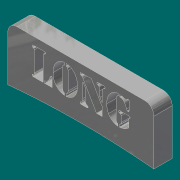
# Autodesk Inventor part: A1-19010-100-04 Tab - LONG
Saved by Autodesk Inventor 2017 SP1 (Build 210196100, 196)
## iProperties
Created: 2014-10-23
Part Number: A1-19010-100-04 Tab - LONG
Material: Steel, Mild
Description: 4" x 1 1/2" x 1/2" PLATE, A516 Gr.70
Document SubType Name: Modeling
Designer: Graeme_Van_Dongen
Density: 7.86 g/cm^3
Appearance: Steel
Mass: 297.606 g
Surface Area: 145.562 cm^2
Volume: 37.8634 cm^3
Author: Graeme_Van_Dongen
Autodesk Inventor part; units mm, degrees
ref_plane "YZ Plane" through (0, 0, 0) normal (1, 0, 0) x (0, 1, 0)
ref_plane "XZ Plane" through (0, 0, 0) normal (0, 1, 0) x (-1, 0, 0)
ref_plane "XY Plane" through (0, 0, 0) normal (0, 0, 1) x (1, 0, 0)
sketch "Sketch1" plane through (0, 0, 0) normal (0, 0, 1) x (1, 0, 0)
  arc A0 (50.8, 543.7321) -> (-50.8, 543.7321) centre (0, 0) ccw
  line L0 (50.8, 543.7321) -> (50.8, 581.8321)
  line L1 (50.8, 581.8321) -> (-50.8, 581.8321)
  line L2 (-50.8, 581.8321) -> (-50.8, 543.7321)
  point P0 (0, 581.8321)
  dimension "d0" = 101.6
  dimension "d1" = 38.1
  dimension "d2" = 546.1
  constraints: 6 end point, 2 parallel, 2 point on circle, 1 centre point, 1 coincident, 1 midpoint, 1 perpendicular, 1 vertical, 1 vertical alignment
  measures "d0" distance of L0.end L1.end
  measures "d1" distance of L0.start L0.end
  measures "d2" radius of A0
extrude "Extrusion1" add sketch "Sketch1" along normal mid plane 12.7
sketch "Sketch2" plane through (0, 0, 6.35) normal (0, 0, 1) x (1, 0, 0)
  line L0 (-46.29, 576.8125) -> (46.3638, 576.8125) construction
  line L1 (46.3638, 576.8125) -> (46.3638, 557.0018) construction
  line L2 (46.3638, 557.0018) -> (-46.29, 557.0018) construction
  line L3 (-46.29, 557.0018) -> (-46.29, 576.8125) construction
  line L4 (-26.3305, 557.3821) -> (-32.5482, 557.3821)
  line L5 (-32.5482, 557.3821) -> (-32.912, 557.3821)
  spline S0 degree 2 poles (-32.912, 557.3821) (-33.4081, 557.3821) (-33.9538, 557.7625) (-33.9538, 558.1097) knots 0 0 0 1 2 2 2
  spline S1 degree 2 poles (-33.9538, 558.1097) (-33.9538, 558.672) (-33.3915, 558.8539) knots 0 0 0 1 1 1
  spline S2 degree 2 poles (-33.3915, 558.8539) (-32.9285, 559.0192) (-32.7797, 559.0854) (-32.697, 559.2177) knots 0 0 0 1 2 2 2
  spline S3 degree 2 poles (-32.697, 559.2177) (-32.5316, 559.4326) (-32.5316, 559.9287) knots 0 0 0 1 1 1
  line L6 (-32.5316, 559.9287) -> (-32.5316, 573.8855)
  spline S4 degree 2 poles (-32.5316, 573.8855) (-32.5316, 574.3816) (-32.697, 574.5966) knots 0 0 0 1 1 1
  spline S5 degree 2 poles (-32.697, 574.5966) (-32.7797, 574.7289) (-32.9285, 574.795) (-33.3915, 574.9438) knots 0 0 0 1 2 2 2
  spline S6 degree 2 poles (-33.3915, 574.9438) (-33.9538, 575.1257) (-33.9538, 575.7045) knots 0 0 0 1 1 1
  spline S7 degree 2 poles (-33.9538, 575.7045) (-33.9538, 576.0518) (-33.4081, 576.4321) (-32.912, 576.4321) knots 0 0 0 1 2 2 2
  line L7 (-32.912, 576.4321) -> (-32.5482, 576.4321)
  line L8 (-32.5482, 576.4321) -> (-26.3139, 576.4321)
  line L9 (-26.3139, 576.4321) -> (-25.8344, 576.4321)
  spline S8 degree 2 poles (-25.8344, 576.4321) (-25.2225, 576.4321) (-24.9579, 576.2667) knots 0 0 0 1 1 1
  spline S9 degree 2 poles (-24.9579, 576.2667) (-24.5941, 576.0352) (-24.5941, 575.6714) knots 0 0 0 1 1 1
  spline S10 degree 2 poles (-24.5941, 575.6714) (-24.5941, 575.0596) (-25.2721, 574.9108) knots 0 0 0 1 1 1
  spline S11 degree 2 poles (-25.2721, 574.9108) (-25.8178, 574.7785) (-26.0163, 574.6958) (-26.1155, 574.58) knots 0 0 0 1 2 2 2
  spline S12 degree 2 poles (-26.1155, 574.58) (-26.3305, 574.3154) (-26.3305, 573.7863) knots 0 0 0 1 1 1
  line L10 (-26.3305, 573.7863) -> (-26.3305, 557.3821)
  line L11 (-25.1895, 557.3821) -> (-25.1895, 558.9531)
  spline S13 degree 2 poles (-25.1895, 558.9531) (-24.5115, 559.0688) (-23.7177, 559.383) (-23.3539, 559.6641) knots 0 0 0 1 2 2 2
  spline S14 degree 2 poles (-23.3539, 559.6641) (-22.7586, 560.1272) (-21.7829, 561.7477) (-21.4853, 562.7399) knots 0 0 0 1 2 2 2
  spline S15 degree 2 poles (-21.4853, 562.7399) (-21.2538, 563.5006) (-20.89, 563.9967) (-20.5262, 563.9967) knots 0 0 0 1 2 2 2
  spline S16 degree 2 poles (-20.5262, 563.9967) (-20.1293, 563.9967) (-19.9474, 563.6825) knots 0 0 0 1 1 1
  spline S17 degree 2 poles (-19.9474, 563.6825) (-19.8647, 563.5171) (-19.8647, 563.0541) knots 0 0 0 1 1 1
  line L12 (-19.8647, 563.0541) -> (-19.8647, 557.3821)
  line L13 (-19.8647, 557.3821) -> (-25.1895, 557.3821)
  line L14 (-10.2405, 575.3076) -> (-10.2405, 576.8125)
  spline S18 degree 2 poles (-10.2405, 576.8125) (-8.7357, 576.7463) (-6.2387, 575.6549) (-5.1638, 574.5966) knots 0 0 0 1 2 2 2
  spline S19 degree 2 poles (-5.1638, 574.5966) (-2.3195, 571.8184) (-2.3195, 566.8906) knots 0 0 0 1 1 1
  spline S20 degree 2 poles (-2.3195, 566.8906) (-2.3195, 562.0454) (-5.0315, 559.3334) knots 0 0 0 1 1 1
  spline S21 degree 2 poles (-5.0315, 559.3334) (-7.1316, 557.2498) (-10.2405, 557.0018) knots 0 0 0 1 1 1
  line L15 (-10.2405, 557.0018) -> (-10.2405, 558.5397)
  spline S22 degree 2 poles (-10.2405, 558.5397) (-9.8767, 558.6223) (-9.4798, 558.8869) (-9.3145, 559.135) knots 0 0 0 1 2 2 2
  spline S23 degree 2 poles (-9.3145, 559.135) (-8.9341, 559.7138) (-8.9341, 560.8713) knots 0 0 0 1 1 1
  line L16 (-8.9341, 560.8713) -> (-8.9341, 573.3398)
  spline S24 degree 2 poles (-8.9341, 573.3398) (-8.9341, 574.0839) (-9.1822, 574.5139) knots 0 0 0 1 1 1
  spline S25 degree 2 poles (-9.1822, 574.5139) (-9.3475, 574.8115) (-9.8105, 575.1423) (-10.2405, 575.3076) knots 0 0 0 1 2 2 2
  spline S26 degree 2 poles (-11.3815, 575.3076) (-12.0926, 575.0431) (-12.6714, 574.1832) (-12.6714, 573.3398) knots 0 0 0 1 2 2 2
  line L17 (-12.6714, 573.3398) -> (-12.6714, 560.8713)
  spline S27 degree 2 poles (-12.6714, 560.8713) (-12.6714, 559.6476) (-12.3406, 559.135) knots 0 0 0 1 1 1
  spline S28 degree 2 poles (-12.3406, 559.135) (-12.076, 558.7216) (-11.3815, 558.5397) knots 0 0 0 1 1 1
  line L18 (-11.3815, 558.5397) -> (-11.3815, 557.0018)
  spline S29 degree 2 poles (-11.3815, 557.0018) (-14.4738, 557.2498) (-16.574, 559.3334) knots 0 0 0 1 1 1
  spline S30 degree 2 poles (-16.574, 559.3334) (-19.2859, 562.0454) (-19.2859, 566.8906) knots 0 0 0 1 1 1
  spline S31 degree 2 poles (-19.2859, 566.8906) (-19.2859, 569.3214) (-17.8473, 573.2406) (-16.4417, 574.5966) knots 0 0 0 1 2 2 2
  spline S32 degree 2 poles (-16.4417, 574.5966) (-15.3668, 575.6549) (-12.8863, 576.7463) (-11.3815, 576.8125) knots 0 0 0 1 2 2 2
  line L19 (-11.3815, 576.8125) -> (-11.3815, 575.3076)
  line L20 (7.3047, 576.4321) -> (14.7296, 563.5337)
  line L21 (14.7296, 563.5337) -> (14.7296, 557.3821)
  line L22 (14.7296, 557.3821) -> (10.9262, 557.3821)
  line L23 (10.9262, 557.3821) -> (1.4508, 573.7036)
  spline S33 degree 2 poles (1.4508, 573.7036) (1.1366, 574.2493) (0.7397, 574.6627) (0.4421, 574.7619) knots 0 0 0 1 2 2 2
  line L24 (0.4421, 574.7619) -> (-0.0871, 574.9604)
  spline S34 degree 2 poles (-0.0871, 574.9604) (-0.3021, 575.0265) (-0.5501, 575.3903) (-0.5501, 575.6053) knots 0 0 0 1 2 2 2
  spline S35 degree 2 poles (-0.5501, 575.6053) (-0.5501, 575.8533) (-0.3021, 576.2502) (-0.0871, 576.3329) knots 0 0 0 1 2 2 2
  spline S36 degree 2 poles (-0.0871, 576.3329) (0.1444, 576.4321) (1.2027, 576.4321) knots 0 0 0 1 1 1
  line L25 (1.2027, 576.4321) -> (7.3047, 576.4321)
  line L26 (1.4508, 571.5208) -> (2.9225, 569.0734)
  line L27 (2.9225, 569.0734) -> (2.9225, 561.5989)
  spline S37 degree 2 poles (2.9225, 561.5989) (2.9225, 560.6233) (3.584, 559.3665) (4.295, 558.9531) knots 0 0 0 1 2 2 2
  line L28 (4.295, 558.9531) -> (4.7085, 558.7216)
  spline S38 degree 2 poles (4.7085, 558.7216) (5.0723, 558.5066) (5.0723, 558.0932) knots 0 0 0 1 1 1
  spline S39 degree 2 poles (5.0723, 558.0932) (5.0723, 557.779) (4.8077, 557.564) knots 0 0 0 1 1 1
  spline S40 degree 2 poles (4.8077, 557.564) (4.5762, 557.3821) (3.8816, 557.3821) knots 0 0 0 1 1 1
  line L29 (3.8816, 557.3821) -> (0.6736, 557.3821)
  spline S41 degree 2 poles (0.6736, 557.3821) (-0.5997, 557.3821) (-0.5997, 558.1097) knots 0 0 0 1 1 1
  spline S42 degree 2 poles (-0.5997, 558.1097) (-0.5997, 558.3578) (-0.3352, 558.6554) (0.1113, 558.9035) knots 0 0 0 1 2 2 2
  spline S43 degree 2 poles (0.1113, 558.9035) (1.4508, 559.6476) (1.4508, 561.5989) knots 0 0 0 1 1 1
  line L30 (1.4508, 561.5989) -> (1.4508, 571.5208)
  line L31 (14.7296, 565.7661) -> (13.2578, 568.2631)
  line L32 (13.2578, 568.2631) -> (13.2578, 572.1326)
  spline S44 degree 2 poles (13.2578, 572.1326) (13.2578, 573.3067) (12.5798, 574.547) (11.7034, 574.9934) knots 0 0 0 1 2 2 2
  spline S45 degree 2 poles (11.7034, 574.9934) (11.4223, 575.1257) (11.1908, 575.4565) (11.1908, 575.7045) knots 0 0 0 1 2 2 2
  spline S46 degree 2 poles (11.1908, 575.7045) (11.1908, 576.0848) (11.6868, 576.4321) (12.2325, 576.4321) knots 0 0 0 1 2 2 2
  line L33 (12.2325, 576.4321) -> (15.7052, 576.4321)
  spline S47 degree 2 poles (15.7052, 576.4321) (16.4163, 576.4321) (16.6478, 576.2006) knots 0 0 0 1 1 1
  spline S48 degree 2 poles (16.6478, 576.2006) (16.8793, 575.9856) (16.8793, 575.6714) knots 0 0 0 1 1 1
  spline S49 degree 2 poles (16.8793, 575.6714) (16.8793, 575.3903) (16.6147, 575.0927) (16.1186, 574.8446) knots 0 0 0 1 2 2 2
  spline S50 degree 2 poles (16.1186, 574.8446) (15.3745, 574.4643) (14.9941, 573.6871) knots 0 0 0 1 1 1
  spline S51 degree 2 poles (14.9941, 573.6871) (14.7296, 573.1083) (14.7296, 572.1326) knots 0 0 0 1 1 1
  line L34 (14.7296, 572.1326) -> (14.7296, 565.7661)
  line L35 (25.8586, 576.8125) -> (25.8586, 575.258)
  spline S52 degree 2 poles (25.8586, 575.258) (24.6349, 574.9604) (24.6349, 573.3067) knots 0 0 0 1 1 1
  line L36 (24.6349, 573.3067) -> (24.6349, 560.3091)
  spline S53 degree 2 poles (24.6349, 560.3091) (24.6349, 559.5649) (24.8499, 559.1515) knots 0 0 0 1 1 1
  spline S54 degree 2 poles (24.8499, 559.1515) (25.0318, 558.8208) (25.6105, 558.5893) knots 0 0 0 1 1 1
  line L37 (25.6105, 558.5893) -> (25.6105, 557.0018)
  spline S55 degree 2 poles (25.6105, 557.0018) (25.1641, 557.0018) (24.4199, 557.1506) (23.8081, 557.349) knots 0 0 0 1 2 2 2
  spline S56 degree 2 poles (23.8081, 557.349) (22.3529, 557.8617) (19.9716, 559.9287) (19.2109, 561.3674) knots 0 0 0 1 2 2 2
  spline S57 degree 2 poles (19.2109, 561.3674) (18.0203, 563.5998) (18.0203, 566.6756) knots 0 0 0 1 1 1
  spline S58 degree 2 poles (18.0203, 566.6756) (18.0203, 569.6522) (20.137, 574.2493) (22.1214, 575.5722) knots 0 0 0 1 2 2 2
  spline S59 degree 2 poles (22.1214, 575.5722) (23.2624, 576.3329) (24.5687, 576.6636) knots 0 0 0 1 1 1
  spline S60 degree 2 poles (24.5687, 576.6636) (25.1144, 576.8125) (25.8586, 576.8125) knots 0 0 0 1 1 1
  spline S61 degree 2 poles (33.3, 559.7138) (32.7378, 559.1515) (30.8857, 557.994) (30.0589, 557.6632) knots 0 0 0 1 2 2 2
  spline S62 degree 2 poles (30.0589, 557.6632) (29.3147, 557.3656) (27.4792, 557.0018) (26.7846, 557.0018) knots 0 0 0 1 2 2 2
  line L38 (26.7846, 557.0018) -> (26.7846, 558.5893)
  spline S63 degree 2 poles (26.7846, 558.5893) (27.198, 558.672) (27.5949, 558.9531) (27.7437, 559.2177) knots 0 0 0 1 2 2 2
  spline S64 degree 2 poles (27.7437, 559.2177) (27.9753, 559.6476) (27.9753, 560.3091) knots 0 0 0 1 1 1
  line L39 (27.9753, 560.3091) -> (27.9753, 564.3936)
  spline S65 degree 2 poles (27.9753, 564.3936) (27.9753, 564.9393) (27.7603, 565.1708) knots 0 0 0 1 1 1
  spline S66 degree 2 poles (27.7603, 565.1708) (27.6611, 565.3031) (27.4792, 565.3858) (26.9335, 565.5015) knots 0 0 0 1 2 2 2
  spline S67 degree 2 poles (26.9335, 565.5015) (26.2555, 565.6669) (26.2555, 566.2787) knots 0 0 0 1 1 1
  spline S68 degree 2 poles (26.2555, 566.2787) (26.2555, 566.6425) (26.8839, 567.0394) (27.4957, 567.0394) knots 0 0 0 1 2 2 2
  line L40 (27.4957, 567.0394) -> (27.9587, 567.0394)
  line L41 (27.9587, 567.0394) -> (33.0685, 567.0394)
  spline S69 degree 2 poles (33.0685, 567.0394) (33.6969, 567.0394) (34.2095, 566.6921) (34.2095, 566.2622) knots 0 0 0 1 2 2 2
  spline S70 degree 2 poles (34.2095, 566.2622) (34.2095, 565.9976) (33.9945, 565.6503) (33.7134, 565.4519) knots 0 0 0 1 2 2 2
  spline S71 degree 2 poles (33.7134, 565.4519) (33.4323, 565.2535) (33.3, 564.9227) (33.3, 564.4763) knots 0 0 0 1 2 2 2
  line L42 (33.3, 564.4763) -> (33.3, 559.7138)
  line L43 (26.9996, 575.2911) -> (26.9996, 576.7959)
  spline S72 degree 2 poles (26.9996, 576.7959) (29.2651, 576.5809) (30.7368, 575.9526) knots 0 0 0 1 1 1
  spline S73 degree 2 poles (30.7368, 575.9526) (31.1668, 575.7541) (31.3983, 575.7541) knots 0 0 0 1 1 1
  spline S74 degree 2 poles (31.3983, 575.7541) (31.6298, 575.7541) (31.8613, 575.9691) (32.2251, 576.4652) knots 0 0 0 1 2 2 2
  spline S75 degree 2 poles (32.2251, 576.4652) (32.4732, 576.8125) (32.8535, 576.8125) knots 0 0 0 1 1 1
  spline S76 degree 2 poles (32.8535, 576.8125) (33.2504, 576.8125) (33.5646, 576.3825) (33.5646, 575.8699) knots 0 0 0 1 2 2 2
  line L44 (33.5646, 575.8699) -> (33.5646, 570.4459)
  spline S77 degree 2 poles (33.5646, 570.4459) (33.5646, 569.371) (32.7874, 569.371) knots 0 0 0 1 1 1
  spline S78 degree 2 poles (32.7874, 569.371) (32.3905, 569.371) (32.0102, 569.7845) (31.8448, 570.4128) knots 0 0 0 1 2 2 2
  spline S79 degree 2 poles (31.8448, 570.4128) (31.6464, 571.1901) (30.5549, 573.2737) (30.0589, 573.869) knots 0 0 0 1 2 2 2
  spline S80 degree 2 poles (30.0589, 573.869) (29.4801, 574.58) (28.0579, 575.225) (26.9996, 575.2911) knots 0 0 0 1 2 2 2
  point P0 (0, 0)
  constraints: 2 other
extrude "Extrusion2" cut sketch "Sketch2" against normal through all
fillet "Fillet1" radius 6.35 2 edges at (-50.8, 581.8321, 0) (50.8, 581.8321, 0)
body "Solid1"
